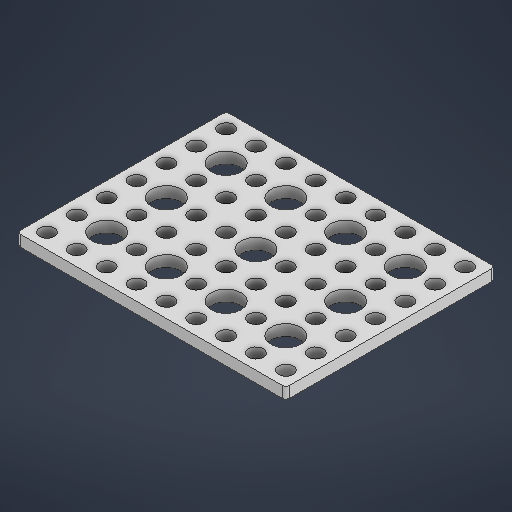
# Autodesk Inventor part: Aluminum Plate
Saved by Autodesk Inventor 2026.1 (Build 301233020, 233B)
## iProperties
Created: 2025-10-19
Part Number: Aluminum Plate
Material: Generic
Document SubType Name: Modeling
Designer: Fennic_zo
Density: 1 g/cm^3
Appearance: Default
Author: Fennic_zo
Autodesk Inventor part; units mm, degrees
ref_plane "YZ Plane" through (0, 0, 0) normal (1, 0, 0) x (0, 1, 0)
ref_plane "XZ Plane" through (0, 0, 0) normal (0, 1, 0) x (-1, 0, 0)
ref_plane "XY Plane" through (0, 0, 0) normal (0, 0, 1) x (1, 0, 0)
sketch "Sketch1" plane through (0, 0, 0) normal (0, 1, 0) x (-1, 0, 0)
  line L0 (0, 0) -> (-72, 0)
  line L1 (-72, 0) -> (-72, -56)
  line L2 (-72, -56) -> (0, -56)
  line L3 (0, -56) -> (0, 0)
  constraints: 8 end point, 2 parallel, 1 horizontal, 1 perpendicular
extrude "Extrusion1" add sketch "Sketch1" along normal blind 3
sketch "Sketch2" plane through (0, 3, 0) normal (0, 1, 0) x (1, 0, 0)
  circle A0 centre (12, 44) radius 4
  line L0 (0, 56) -> (0, 0) projected
  line L1 (72, 56) -> (0, 56) projected
  circle A1 centre (12, 28) radius 4
  circle A2 centre (12, 12) radius 4
  circle A3 centre (28, 44) radius 4
  circle A4 centre (28, 12) radius 4
  circle A5 centre (44, 44) radius 4
  circle A6 centre (44, 12) radius 4
  circle A7 centre (60, 44) radius 4
  circle A8 centre (60, 12) radius 4
  circle A9 centre (60, 28) radius 4
  circle A10 centre (36, 28) radius 4
  circle A11 centre (4, 52) radius 2
  circle A12 centre (12, 52) radius 2
  circle A13 centre (20, 52) radius 2
  circle A14 centre (28, 52) radius 2
  circle A15 centre (36, 52) radius 2
  circle A16 centre (44, 52) radius 2
  circle A17 centre (52, 52) radius 2
  circle A18 centre (60, 52) radius 2
  circle A19 centre (68, 52) radius 2
  circle A20 centre (4, 44) radius 2
  circle A21 centre (4, 36) radius 2
  circle A22 centre (4, 28) radius 2
  circle A23 centre (4, 20) radius 2
  circle A24 centre (4, 12) radius 2
  circle A25 centre (4, 4) radius 2
  circle A26 centre (12, 4) radius 2
  circle A27 centre (20, 4) radius 2
  circle A28 centre (28, 4) radius 2
  circle A29 centre (36, 4) radius 2
  circle A30 centre (44, 4) radius 2
  circle A31 centre (52, 4) radius 2
  circle A32 centre (60, 4) radius 2
  circle A33 centre (68, 4) radius 2
  circle A34 centre (68, 44) radius 2
  circle A35 centre (68, 36) radius 2
  circle A36 centre (68, 28) radius 2
  circle A37 centre (68, 20) radius 2
  circle A38 centre (68, 12) radius 2
  circle A39 centre (68, 4) radius 2
  circle A40 centre (12, 36) radius 2
  circle A41 centre (20, 36) radius 2
  circle A42 centre (28, 36) radius 2
  circle A43 centre (36, 36) radius 2
  circle A44 centre (44, 36) radius 2
  circle A45 centre (52, 36) radius 2
  circle A46 centre (60, 36) radius 2
  circle A47 centre (12, 20) radius 2
  circle A48 centre (20, 20) radius 2
  circle A49 centre (28, 20) radius 2
  circle A50 centre (36, 20) radius 2
  circle A51 centre (44, 20) radius 2
  circle A52 centre (52, 20) radius 2
  circle A53 centre (60, 20) radius 2
  circle A54 centre (20, 44) radius 2
  circle A55 centre (36, 44) radius 2
  circle A56 centre (52, 44) radius 2
  circle A57 centre (20, 12) radius 2
  circle A58 centre (36, 12) radius 2
  circle A59 centre (52, 12) radius 2
  circle A60 centre (20, 28) radius 2
  circle A61 centre (28, 28) radius 2
  circle A62 centre (44, 28) radius 2
  circle A63 centre (52, 28) radius 2
  dimension "d2" = 8
  dimension "d3" = 8
  dimension "d4" = 8
  dimension "d7" = 16
  dimension "d14" = 16
  dimension "d21" = 16
  dimension "d28" = 24
  dimension "d33" = 4
  dimension "d34" = 2
  dimension "d35" = 2
  dimension "d38" = 8
  dimension "d45" = 8
  dimension "d52" = 8
  dimension "d59" = 8
  dimension "d66" = 8
  dimension "d73" = 8
  dimension "d80" = 8
  dimension "d87" = 8
  dimension "d94" = 8
  constraints: 64 centre point, 7 vertical, 6 horizontal, 124 other
  measures "d2" distance edge to line of A0 L0
  measures "d3" diameter of A0
  measures "d4" distance edge to line of A0 L1
  measures "d7" distance of A0.centre A1.centre
  measures "d14" distance of A0.centre A3.centre
  measures "d21" distance of A7.centre A9.centre
  measures "d28" distance of A1.centre A10.centre
  measures "d33" diameter of A11
  measures "d34" distance edge to line of A11 L1
  measures "d35" distance edge to line of A11 L0
  measures "d38" distance of A11.centre A12.centre
  measures "d45" distance of A11.centre A20.centre
  measures "d52" distance of A25.centre A26.centre
  measures "d59" distance of A19.centre A34.centre
  measures "d66" distance of A21.centre A40.centre
  measures "d73" distance of A23.centre A47.centre
  measures "d80" distance of A13.centre A54.centre
  measures "d87" distance of A27.centre A57.centre
  measures "d94" distance of A48.centre A60.centre
fillet "Fillet1" radius 1 4 edges at (72, 1.5, -56) (72, 1.5, 0) (0, 1.5, 0) (0, 1.5, -56)
extrude "Extrusion2" cut sketch "Sketch2" against normal blind 4
body "Solid1"
